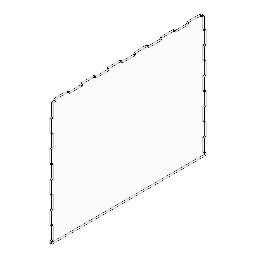
Sides v5 (Autodesk Fusion 360 design; units mm, degrees)
Autodesk Fusion 360 part; units mm, degrees
sketch "Sketch1" plane through (0, 0, 0) normal (1, 0, 0) x (0, 1, 0)
  line L0 (0, 0) -> (350, 0)
  line L1 (350, 0) -> (350, 280)
  line L2 (350, 280) -> (0, 280)
  line L3 (0, 280) -> (0, 0)
  line L4 (0, 276) -> (4, 276)
  line L5 (4, 276) -> (4, 246)
  line L6 (4, 246) -> (0, 246)
  line L7 (0, 246) -> (0, 276)
  line L8 (40, 280) -> (70, 280)
  line L9 (70, 280) -> (70, 276)
  line L10 (70, 276) -> (40, 276)
  line L11 (40, 276) -> (40, 280)
  line L12 (0, 280) -> (10, 280)
  line L13 (10, 280) -> (10, 276)
  line L14 (10, 276) -> (0, 276)
  line L15 (0, 276) -> (0, 280)
  dimension "d5" = 350
  dimension "d6" = 280
  dimension "d7" = 30
  dimension "d8" = 30
  dimension "d9" = 4
  dimension "d10" = 4
  dimension "d14" = 10
  dimension "d15" = 4
  dimension "d16" = 30
  constraint horizontal L0
  constraint vertical L1
  constraint horizontal L2
  constraint vertical L3
  constraint coincident L0.start L3.end
  constraint horizontal L4
  constraint vertical L5
  constraint horizontal L6
  constraint vertical L7
  constraint coincident L3 L4.start
  constraint horizontal L8
  constraint vertical L9
  constraint horizontal L10
  constraint vertical L11
  constraint coincident L2 L8.start
  constraint horizontal L12
  constraint vertical L13
  constraint vertical L15
  constraint coincident L4.end L14
  measures "d5" distance of L0.start L0.end
  measures "d6" distance of L0.start L2.end
  measures "d7" distance of L4.end L5.end
  measures "d8" distance of L9.end L10.end
  measures "d9" distance of L8.end L9.end
  measures "d10" distance of L5.end L6.end
  measures "d14" distance of L13.end L4.start
  measures "d15" distance of L12.end L13.end
  measures "d16" distance of L10.end L13.end
extrude "Extrude1" add sketch "Sketch1" along normal blind 4 makes body 1
extrude "Extrude2" cut sketch "Sketch1" along normal through all contours L3 L4 L5 L6 L7 L14 bodies 1
extrude "Extrude3" cut sketch "Sketch1" along normal through all contours L2 L3 L4 L12 L13 L14 L15 bodies 1
extrude "Extrude4" cut sketch "Sketch1" along normal through all contours L2 L8 L9 L10 L11 bodies 1
pattern_linear "R-Pattern1" count 5 spacing 60 along (0, 0, -1) count 2 spacing 346 along (0, 1, 0) of "Extrude2"
pattern_linear "R-Pattern2" count 2 spacing 340 along (0, 1, 0) of "Extrude3"
pattern_linear "R-Pattern3" count 5 spacing 60 along (0, 1, 0) of "Extrude4"
copy_body "Body->Comp1" bodies 1 removing the originals makes body 2 in component "Component"
component "Component" placed x (1, 0, 0) y (0, 1, 0) z (0, 0, 1) at (0, 0, 0)
equation "d = 350 mm"
equation "h = 280 mm"
equation "a = 30 mm"
equation "t = 4 mm"
equation "d5 = d"
equation "d6 = h"
equation "d9 = t"
equation "d10 = t"
equation "a_d = ( d - floor(d / a) * a ) / 2"
equation "d14 = a_d"
equation "d15 = t"
equation "d16 = a"
equation "d17 = t"
equation "n_h = floor(floor(h / a) / 2) + 1"
equation "n_d = floor(floor(d / a) / 2)"
equation "d25 = n_h"
equation "d27 = a * 2"
equation "d28 = d - t"
equation "d31 = d - a_d"
equation "d33 = n_d"
equation "d35 = 2 * a"
